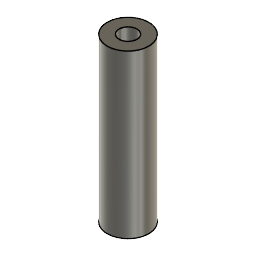
track_rod (Autodesk Fusion 360 design; units mm, degrees)
part number: 2026-03-06-16-14-00-828
Autodesk Fusion 360 part; units mm, degrees
sketch "Skizze1" plane through (0, 0, 0) normal (0, 0, 1) x (1, 0, 0)
  circle A0 centre (3, -3) radius 0.99
  circle A1 centre (3, -3) radius 2.3
  dimension "d3" = 1.98
  dimension "d11" = 4.6
  constraint concentric A0 A1
  measures "d3" diameter of A0
  measures "d11" diameter of A1
extrude "Extrusion1" add sketch "Skizze1" along normal blind 18
equation "d3 = 1.8 * 1.1 mm"
named bodies: "Track Rod"
